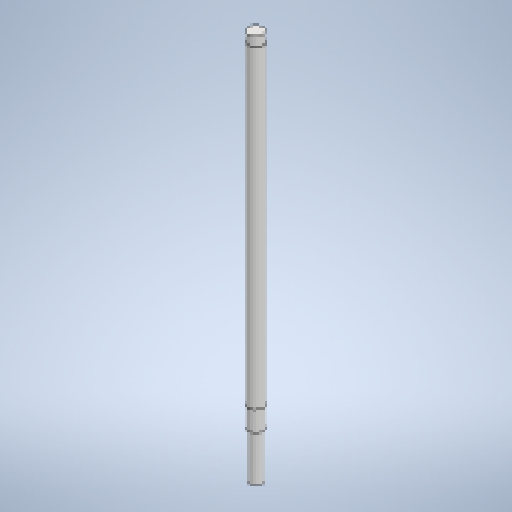
# Autodesk Inventor part: TRM 028 main shaft
Saved by Autodesk Inventor 2025 (Build 290162010, 162A)
## iProperties
Created: 2024-09-08
Part Number: TRM 028 main shaft
Material: Generic
Document SubType Name: Modeling
Designer: admin
Density: 1 g/cm^3
Appearance: Default
Mass: 304.342 g
Surface Area: 496.764 cm^2
Volume: 304.342 cm^3
Author: admin
Autodesk Inventor part; units mm, degrees
ref_plane "YZ Plane" through (0, 0, 0) normal (1, 0, 0) x (0, 1, 0)
ref_plane "XZ Plane" through (0, 0, 0) normal (0, 1, 0) x (-1, 0, 0)
ref_plane "XY Plane" through (0, 0, 0) normal (0, 0, 1) x (1, 0, 0)
sketch "Sketch1" plane through (0, 0, 0) normal (0, 1, 0) x (-1, 0, 0)
  line L0 (0, 0) -> (0, 280)
  line L1 (0, 280) -> (-12.5, 280)
  line L2 (-12.5, 280) -> (-12.5, 0)
  line L3 (-12.5, 0) -> (-12.5, -390)
  line L4 (-12.5, -390) -> (0, -390)
  line L5 (0, -390) -> (0, 0)
  line L6 (-9.5, -390) -> (-9.5, -310)
  line L7 (-9.5, -310) -> (-12.5, -310)
  line L8 (-12.5, -275) -> (-12, -275)
  line L9 (-12, -275) -> (-12, -310)
  line L10 (-12, 280) -> (-12, 265)
  line L11 (-12, 265) -> (-12.5, 265)
  dimension "d0" = 25
  dimension "d1" = 280
  dimension "d2" = 390
  dimension "d4" = 80
  dimension "d5" = 19
  dimension "d6" = 24
  dimension "d7" = 35
  dimension "d8" = 15
  constraints: 24 end point, 9 perpendicular, 8 point on line, 1 collinear, 1 horizontal alignment, 1 parallel, 1 vertical
  measures "d0" diameter of L2 L0
  measures "d1" distance of L1.end L2.end
  measures "d2" distance of L2.end L3.end
  measures "d4" distance of L6.start L6.end
  measures "d5" diameter of L6 L5
  measures "d6" diameter of L9 L5
  measures "d7" distance of L8.end L9.end
  measures "d8" distance of L10.start L10.end
revolve "Revolution1" add sketch "Sketch1" angle 360 about axis through (0, 0, 0) along (0, 0, 1) contours L5 L4 L6 L7 L9 L8 L3 L2 L11 L10 L1 L0
body "Solid1"
